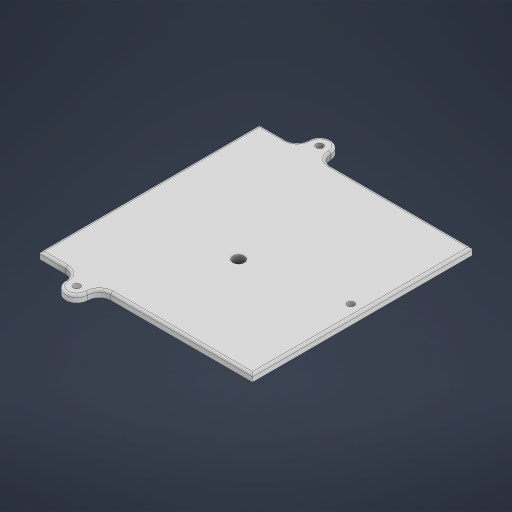
# Autodesk Inventor part: Cover
Saved by Autodesk Inventor 2024.2 (Build 282272000, 272)
## iProperties
Created: 2024-03-13
Part Number: Cover
Material: Generic
Document SubType Name: Modeling
Designer: jerem
Density: 1 g/cm^3
Appearance: Default
Author: jerem
## iProperties of the stored document Battery_Cover_3DPrint.ipt
Created: 2024-03-21
Part Number: Battery_Cover_3DPrint
Material: Generic
Document SubType Name: Modeling
Designer: jerem
Density: 1 g/cm^3
Appearance: Default
Author: jerem
Autodesk Inventor part; units mm, degrees
ref_plane "YZ Plane" through (0, 0, 0) normal (1, 0, 0) x (0, 1, 0)
ref_plane "XZ Plane" through (0, 0, 0) normal (0, 1, 0) x (-1, 0, 0)
ref_plane "XY Plane" through (0, 0, 0) normal (0, 0, 1) x (1, 0, 0)
sketch "Sketch1" plane through (0, 0, 0) normal (0, 1, 0) x (-1, 0, 0)
  line L0 (-46, -47.5) -> (46, -47.5)
  line L1 (46, -47.5) -> (46, 47.5)
  line L2 (46, 47.5) -> (-46, 47.5)
  line L3 (-46, 47.5) -> (-46, -47.5)
  line L4 (-46, -47.5) -> (46, 47.5) construction
  line L5 (46, -47.5) -> (-46, 47.5) construction
  line L6 (46, 0) -> (-46, 0) construction
  circle A0 centre (25, -52.5) radius 1.5
  circle A1 centre (25, -52.5) radius 4.75
  arc A2 (20.25, -52.5) -> (15.25, -47.5) centre (15.25, -52.5) ccw
  arc A3 (34.75, -47.5) -> (29.75, -52.5) centre (34.75, -52.5) ccw
  circle A4 centre (-41, 0) radius 1.5
  circle A5 centre (25, -52.5) radius 3.5
  circle A6 centre (-41, 0) radius 3.5
  line L7 (-46, -47.5) -> (-46, 47.5)
  circle A7 centre (25, 52.5) radius 1.5
  circle A8 centre (25, 52.5) radius 4.75
  arc A9 (15.25, 47.5) -> (20.25, 52.5) centre (15.25, 52.5) ccw
  arc A10 (29.75, 52.5) -> (34.75, 47.5) centre (34.75, 52.5) ccw
  circle A11 centre (25, 52.5) radius 3.5
  point P0 (0, 0)
  point P1 (4.1863, 47.5)
  point P2 (34.75, 47.5)
  point P3 (15.25, 47.5)
  dimension "d2" = 95
  dimension "d101" = 21
  dimension "d102" = 3
  dimension "d103" = 9.5
  dimension "d104" = 5
  dimension "d105" = 5
  dimension "d106" = 5
  dimension "d107" = 3
  dimension "d108" = 5
  dimension "d109" = 92
  dimension "d110" = 7
  dimension "d111" = 7
  constraints: 16 end point, 12 centre point, 12 point on circle, 11 symmetric about line, 5 coincident, 4 midpoint, 4 point on line, 4 tangent, 2 parallel, 1 horizontal, 1 perpendicular, 5 other
  measures "d2" distance of L0.end L1.end
  measures "d101" distance from line of A0.centre L1
  measures "d102" diameter of A0
  measures "d103" diameter of A1
  measures "d104" distance from line of L0 A0.centre
  measures "d105" radius of A2
  measures "d106" radius of A3
  measures "d107" diameter of A4
  measures "d108" distance from line of L3 A4.centre
  measures "d109" distance of L1.end L2.end
  measures "d110" diameter of A5
  measures "d111" diameter of A6
extrude "Extrusion1" add sketch "Sketch1" along normal blind 3 contours L3 L2 L1 L0 | L0 A3 A1 A2 | A1 | A9 A8 A10 L2 | A8 | A5 | A6 | A11
fillet "Fillet1" radius 1 6 edges at (46, 3, 0) (-40.375, 3, -47.5) (15.375, 3, -47.5) (-46, 3, 0) (-40.375, 3, 47.5) (15.375, 3, 47.5) curvature continuous yes
sketch "Sketch3" plane through (0, 0, 0) normal (0, -1, 0) x (1, 0, 0)
  line L0 (-12.25, -0.2123) -> (-12.25, -24.7123)
  line L1 (-12.25, -24.7123) -> (5.25, -24.7123)
  line L2 (5.25, -24.7123) -> (5.25, -21.2123)
  line L3 (5.25, -21.2123) -> (0, -21.2123)
  line L4 (0, -21.2123) -> (0, -17.7123)
  line L5 (0, -17.7123) -> (5.25, -17.7123)
  line L6 (5.25, -17.7123) -> (5.25, -14.2123)
  line L7 (5.25, -14.2123) -> (-3.5, -14.2123)
  line L8 (-3.5, -14.2123) -> (-3.5, -21.2123)
  line L9 (-3.5, -21.2123) -> (-8.75, -21.2123)
  line L10 (-8.75, -21.2123) -> (-8.75, 3.1161)
  line L11 (-12.25, -0.2123) -> (-12.25, 24.7123)
  line L12 (-12.25, 24.7123) -> (-8.75, 24.7123)
  line L13 (-8.75, 24.7123) -> (-8.75, 3.1161)
  line L14 (-5.25, 24.7123) -> (-5.25, 17.7123)
  line L15 (-5.25, 17.7123) -> (-2.7751, 15.2374)
  line L16 (-2.7751, 15.2374) -> (0.7249, 15.2374)
  line L17 (0.7249, 15.2374) -> (3.5, 18.0126)
  line L18 (3.5, 18.0126) -> (6.2751, 15.2374)
  line L19 (6.2751, 15.2374) -> (9.7751, 15.2374)
  line L20 (9.7751, 15.2374) -> (12.25, 17.7123)
  line L21 (12.25, 17.7123) -> (12.25, 24.7123)
  line L22 (12.25, 24.7123) -> (-5.25, 24.7123)
  line L23 (-5.25, 9.2626) -> (-5.25, 5.7626)
  line L24 (-5.25, 9.2626) -> (-2.7751, 11.7374)
  line L25 (-2.7751, 11.7374) -> (2.7751, 11.7374)
  line L26 (12.25, 11.7374) -> (8.75, 11.7374)
  line L27 (8.75, 11.7374) -> (8.75, -0.2123)
  line L28 (8.75, -0.2123) -> (-5.25, -0.2123)
  line L29 (-5.25, -0.2123) -> (-5.25, -3.7123)
  line L30 (-5.25, -3.7123) -> (8.75, -3.7123)
  line L31 (8.75, -3.7123) -> (8.75, -7.2123)
  line L32 (8.75, -7.2123) -> (-5.25, -7.2123)
  line L33 (-5.25, -7.2123) -> (-5.25, -10.7123)
  line L34 (-5.25, -10.7123) -> (8.75, -10.7123)
  line L35 (8.75, -10.7123) -> (8.75, -24.7123)
  line L36 (8.75, -24.7123) -> (12.25, -24.7123)
  line L37 (12.25, -24.7123) -> (12.25, 11.7374)
  line L38 (-5.25, 5.7626) -> (-2.7751, 3.2877)
  line L39 (-5.25, 5.7626) -> (-1.75, 5.7626) construction
  line L40 (-2.7751, 3.2877) -> (2.7751, 3.2877)
  line L41 (2.7751, 3.2877) -> (5.25, 5.7626)
  line L42 (5.25, 5.7626) -> (5.25, 9.2626)
  line L43 (5.25, 9.2626) -> (2.7751, 11.7374)
  line L44 (12.25, -24.7123) -> (46, -24.7123) construction
  line L45 (46, 47.5) -> (46, -47.5) construction
  line L46 (-12.25, -24.7123) -> (-46, -24.7123) construction
  line L47 (-46, -47.5) -> (-46, 47.5) construction
  line L48 (12.25, -24.7123) -> (12.25, -47.5) construction
  line L49 (-34.75, -47.5) -> (-46, -47.5) construction
  line L50 (12.25, 24.7123) -> (12.25, 47.5) construction
  line L51 (-46, 47.5) -> (-34.75, 47.5) construction
  point P0 (0, 0)
  point P1 (2.625, -21.2123)
  point P2 (-5.25, -8.9623)
  point P3 (18.5, 41)
  point P4 (46, -47.5)
  point P5 (-18.5, -41)
  point P6 (7, -41)
  point P7 (7, 41)
  dimension "d61" = 3.5
  dimension "d62" = 3.5
  dimension "d63" = 3.5
  dimension "d64" = 3.5
  dimension "d65" = 3.5
  dimension "d66" = 135
  dimension "d67" = 3.5
  dimension "d68" = 3.5
  dimension "d69" = 3.5
  dimension "d70" = 3.5
  dimension "d71" = 3.5
  dimension "d72" = 3.5
  dimension "d73" = 3.5
  dimension "d74" = 135
  dimension "d75" = 3.5
  dimension "d76" = 3.5
  dimension "d77" = 3.5
  dimension "d78" = 3.5
  dimension "d79" = 45
  dimension "d80" = 3.5
  dimension "d81" = 3.5
  dimension "d82" = 3.5
  dimension "d83" = 3.5
  dimension "d84" = 3.5
  dimension "d85" = 3.5
  dimension "d86" = 3.5
  dimension "d87" = 1.75
  dimension "d88" = 7
  dimension "d89" = 5.25
  dimension "d90" = 3.5
  dimension "d91" = 3.5
  dimension "d92" = 3.5
  dimension "d93" = 3.5
  dimension "d94" = 0
  constraints: 96 end point, 27 perpendicular, 11 point on line, 6 collinear, 5 horizontal, 4 vertical, 3 equal length, 2 midpoint, 1 parallel, 8 other
  measures "d61" distance between parallel lines of L7 L5
  measures "d62" distance between parallel lines of L8 L4
  measures "d63" distance from line of L1 point (2.625, -21.212)
  measures "d64" distance between parallel lines of L9 L1
  measures "d65" distance between parallel lines of L0 L10
  measures "d66" angle of L15 L14
  measures "d67" distance between parallel lines of L32 L30
  measures "d68" distance between parallel lines of L30 L28
  measures "d69" distance between parallel lines of L34 L32
  measures "d70" distance between parallel lines of L35 L37
  measures "d71" distance between parallel lines of L10 L29
  measures "d72" distance between parallel lines of L13 L23
  measures "d73" distance between parallel lines of L25 L16
  measures "d74" angle of L23 L24
  measures "d75" distance between parallel lines of L13 L14
  measures "d76" distance between parallel lines of L35 L6
  measures "d77" distance of L15.end L16.end
  measures "d78" distance of L19.start L19.end
  measures "d79" angle of L38 L39
  measures "d80" distance of L24.start L23.end
  measures "d81" distance between parallel lines of L27 L42
  measures "d82" distance of L42.start L43.start
  measures "d83" distance between parallel lines of L3 L5
  measures "d84" distance between parallel lines of L34 L7
  measures "d85" distance between parallel lines of L40 L28
  measures "d86" distance of L19.end L20.end
  measures "d87" distance from line of point (-5.25, -8.962) L8
  measures "d88" distance of L20.end L22.start
  measures "d89" distance between parallel lines of L4 L2
  measures "d90" distance of L41.start L42.start
  measures "d91" distance of L24.start L25.start
  measures "d92" distance of L23.end L38.end
  measures "d93" distance of L43.start L25.end
  measures "d94" distance from line of L0.start L28
extrude "Extrusion3" add sketch "Sketch3" along normal blind 2
sketch "Sketch2" plane through (0, 0, 0) normal (0, -1, 0) x (1, 0, 0)
  line L0 (0, 0) -> (0, -14)
  line L1 (0, -14) -> (10, -14)
  line L2 (10, -14) -> (10, -12)
  line L3 (10, -12) -> (7, -12)
  line L4 (7, -12) -> (7, -10)
  line L5 (7, -10) -> (10, -10)
  line L6 (10, -10) -> (10, -8)
  line L7 (10, -8) -> (5, -8)
  line L8 (5, -8) -> (5, -12)
  line L9 (5, -12) -> (2, -12)
  line L10 (2, -12) -> (2, 0.5333)
  line L11 (0, 0) -> (0, 14.2426)
  line L12 (0, 14.2426) -> (2, 14.2426)
  line L13 (2, 14.2426) -> (2, 0.5333)
  line L14 (4, 14.2426) -> (4, 10.2426)
  line L15 (4, 10.2426) -> (5.4142, 8.8284)
  line L16 (5.4142, 8.8284) -> (7.4142, 8.8284)
  line L17 (7.4142, 8.8284) -> (9, 10.4142)
  line L18 (9, 10.4142) -> (10.5858, 8.8284)
  line L19 (10.5858, 8.8284) -> (12.5858, 8.8284)
  line L20 (12.5858, 8.8284) -> (14, 10.2426)
  line L21 (14, 10.2426) -> (14, 14.2426)
  line L22 (14, 14.2426) -> (4, 14.2426)
  line L23 (4, 5.4142) -> (4, 3.4142)
  line L24 (4, 5.4142) -> (5.4142, 6.8284)
  line L25 (5.4142, 6.8284) -> (8.5858, 6.8284)
  line L26 (14, 6.8284) -> (12, 6.8284)
  line L27 (12, 6.8284) -> (12, 0)
  line L28 (12, 0) -> (4, 0)
  line L29 (4, 0) -> (4, -2)
  line L30 (4, -2) -> (12, -2)
  line L31 (12, -2) -> (12, -4)
  line L32 (12, -4) -> (4, -4)
  line L33 (4, -4) -> (4, -6)
  line L34 (4, -6) -> (12, -6)
  line L35 (12, -6) -> (12, -14)
  line L36 (12, -14) -> (14, -14)
  line L37 (14, -14) -> (14, 6.8284)
  line L38 (4, 3.4142) -> (5.4142, 2)
  line L39 (4, 3.4142) -> (6, 3.4142) construction
  line L40 (5.4142, 2) -> (8.5858, 2)
  line L41 (8.5858, 2) -> (10, 3.4142)
  line L42 (10, 3.4142) -> (10, 5.4142)
  line L43 (10, 5.4142) -> (8.5858, 6.8284)
  point P0 (8.5, -12)
  point P1 (4, -5)
  dimension "d13" = 2
  dimension "d14" = 2
  dimension "d15" = 2
  dimension "d16" = 2
  dimension "d17" = 2
  dimension "d18" = 135
  dimension "d20" = 2
  dimension "d21" = 2
  dimension "d22" = 2
  dimension "d23" = 2
  dimension "d24" = 2
  dimension "d25" = 2
  dimension "d26" = 2
  dimension "d28" = 135
  dimension "d29" = 2
  dimension "d30" = 2
  dimension "d31" = 2
  dimension "d32" = 2
  dimension "d33" = 45
  dimension "d35" = 2
  dimension "d36" = 2
  dimension "d39" = 2
  dimension "d40" = 2
  dimension "d41" = 2
  dimension "d42" = 2
  dimension "d43" = 2
  dimension "d44" = 1
  dimension "d45" = 4
  dimension "d50" = 3
  dimension "d51" = 2
  dimension "d52" = 2
  dimension "d53" = 2
  dimension "d54" = 2
  dimension "d55" = 0
  constraints: 88 end point, 27 perpendicular, 9 point on line, 6 collinear, 4 horizontal, 3 vertical, 2 midpoint, 1 equal length, 1 parallel
  measures "d13" distance between parallel lines of L7 L5
  measures "d14" distance between parallel lines of L8 L4
  measures "d15" distance from line of L1 point (8.5, -12)
  measures "d16" distance between parallel lines of L9 L1
  measures "d17" distance between parallel lines of L0 L10
  measures "d18" angle of L15 L14
  measures "d20" distance between parallel lines of L32 L30
  measures "d21" distance between parallel lines of L30 L28
  measures "d22" distance between parallel lines of L34 L32
  measures "d23" distance between parallel lines of L35 L37
  measures "d24" distance between parallel lines of L10 L29
  measures "d25" distance between parallel lines of L13 L23
  measures "d26" distance between parallel lines of L25 L16
  measures "d28" angle of L23 L24
  measures "d29" distance between parallel lines of L13 L14
  measures "d30" distance between parallel lines of L35 L6
  measures "d31" distance of L15.end L16.end
  measures "d32" distance of L18.end L19.end
  measures "d33" angle of L38 L39
  measures "d35" distance of L23.start L23.end
  measures "d36" distance between parallel lines of L27 L42
  measures "d39" distance of L41.end L42.end
  measures "d40" distance between parallel lines of L3 L5
  measures "d41" distance between parallel lines of L34 L7
  measures "d42" distance between parallel lines of L40 L28
  measures "d43" distance of L19.end L20.end
  measures "d44" distance from line of point (4, -5) L8
  measures "d45" distance of L20.end L21.end
  measures "d50" distance between parallel lines of L4 L2
  measures "d51" distance of L40.end L41.end
  measures "d52" distance of L23.start L24.end
  measures "d53" distance of L23.end L38.end
  measures "d54" distance of L42.end L25.end
  measures "d55" distance from line of L0.start L28
chamfer "Chamfer2" distance 1.5 angle 45 40 edges at (-5.25, 0, 21.2123) (-4.0126, 0, 16.4749) (-1.0251, 0, 15.2374) (2.1124, 0, 16.625) (4.8876, 0, 16.625) (8.0251, 0, 15.2374) (11.0126, 0, 16.4749) (12.25, 0, 21.2123) (3.5, 0, 24.7123) (-8.75, 0, 1.75) (-10.5, 0, 24.7123) (-12.25, 0, 0) (-3.5, 0, -24.7123) (5.25, 0, -22.9623) (2.625, 0, -21.2123) (0, 0, -19.4623) (2.625, 0, -17.7123) (5.25, 0, -15.9623) (0.875, 0, -14.2123) (-3.5, 0, -17.7123) (8.75, 0, -17.7123) (10.5, 0, -24.7123) (12.25, 0, -6.4874) (1.75, 0, -10.7123) (-5.25, 0, -8.9623) (1.75, 0, -7.2123) (1.75, 0, -3.7123) (1.75, 0, -0.2123) (10.5, 0, 11.7374) (8.75, 0, 5.7626) (5.25, 0, 7.5126) (4.0126, 0, 4.5251) (0, 0, 3.2877) (-4.0126, 0, 4.5251) (-5.25, 0, 7.5126) (-4.0126, 0, 10.5) (0, 0, 11.7374) (4.0126, 0, 10.5) (-5.25, 0, -1.9623) (-6.125, 0, -21.2123)
extrude "Extrusion4" cut sketch "Sketch1" along normal blind 1 contours A4 | A5 | A6 | A11
sketch "Sketch4" plane through (0, -2, 0) normal (0, -1, 0) x (1, 0, 0)
  line L0 (2.7751, 3.2877) -> (5.25, 5.7626) construction
  line L1 (-5.25, 9.2626) -> (-5.25, 5.7626) construction
  line L2 (5.25, 5.7626) -> (-5.25, 9.2626) construction
  line L3 (-5.25, 9.2626) -> (-5.25, 5.7626) construction
  line L4 (5.25, 5.7626) -> (5.25, 9.2626) construction
  line L5 (-5.25, 5.7626) -> (5.25, 9.2626) construction
  circle A0 centre (0, 7.5126) radius 2.5
  point P0 (0, 0)
  dimension "d114" = 5
  constraints: 6 end point, 1 centre point, 1 collinear, 1 midpoint
  measures "d114" diameter of A0
extrude "Extrusion5" cut sketch "Sketch4" against normal up to surface (5 mm away)
equation "\"d14\" = d13"
equation "\"d15\" = d13"
equation "\"d16\" = d13"
equation "\"d17\" = d13"
equation "\"d20\" = d13"
equation "\"d21\" = d13"
equation "\"d22\" = d13"
equation "\"d23\" = d13"
equation "\"d24\" = d13"
equation "\"d25\" = d13"
equation "\"d26\" = d13"
equation "\"d29\" = d13"
equation "\"d30\" = d13"
body "Solid1"
